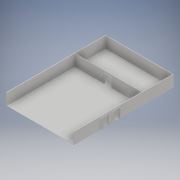
# Autodesk Inventor part: Top Office Layer
Saved by Autodesk Inventor 2017 (Build 210142000, 142)
## iProperties
Created: 2018-04-17
Part Number: Top Office Layer
Material: Generic
Document SubType Name: Modeling
Designer: landontracy
Density: 1 g/cm^3
Appearance: Default
Author: landontracy
Autodesk Inventor part; units mm, degrees
ref_plane "YZ Plane" through (0, 0, 0) normal (1, 0, 0) x (0, 1, 0)
ref_plane "XZ Plane" through (0, 0, 0) normal (0, 1, 0) x (-1, 0, 0)
ref_plane "XY Plane" through (0, 0, 0) normal (0, 0, 1) x (1, 0, 0)
sketch "Sketch1" plane through (0, 0, 0) normal (0, 0, 1) x (1, 0, 0)
  line L0 (-105.4358, -42.0697) -> (85.0642, -42.0697)
  line L1 (85.0642, -42.0697) -> (85.0642, 186.5303)
  line L2 (85.0642, 186.5303) -> (-105.4358, 186.5303)
  line L3 (-105.4358, 186.5303) -> (-105.4358, -42.0697)
  line L4 (-105.4358, -42.0697) -> (-156.2358, -42.0697)
  line L5 (-156.2358, -42.0697) -> (-156.2358, 237.3303)
  line L6 (-156.2358, 237.3303) -> (135.8642, 237.3303)
  line L7 (135.8642, 237.3303) -> (135.8642, -42.0697)
  line L8 (135.8642, -42.0697) -> (85.0642, -42.0697)
  point P0 (0, 0)
  dimension "d0" = 228.6
  dimension "d1" = 190.5
  dimension "d2" = 50.8
  dimension "d3" = 279.4
  dimension "d4" = 292.1
  constraints: 18 end point, 5 perpendicular, 2 horizontal, 2 parallel, 1 point on line
  measures "d0" distance of L0.end L1.end
  measures "d1" distance of L0.start L0.end
  measures "d2" distance of L0.start L4.end
  measures "d3" distance of L4.end L5.end
  measures "d4" distance of L5.end L6.end
extrude "Door Frame CR" add sketch "Sketch1" along normal mid plane 8.89 contours L4 L5 L6 L7 L8 L1 L2 L3
sketch "Sketch2" plane through (-156.2358, -42.0697, 4.445) normal (-1, 0, 0) x (0, 0, 1)
  line L0 (-8.89, 279.4) -> (-8.89, 0) projected
  line L1 (-8.89, 279.4) -> (0, 279.4)
  line L2 (0, 279.4) -> (0, 0)
  line L3 (0, 0) -> (-8.89, 0)
  line L4 (-8.89, 0) -> (-8.89, 279.4)
  point P0 (-4.445, 42.0697)
  constraints: 8 end point, 2 parallel, 1 horizontal, 1 perpendicular
extrude "Door Frame left Extruded" add sketch "Sketch2" along normal blind 685.8
sketch "Sketch4" plane through (135.8642, -42.0697, 4.445) normal (1, 0, 0) x (0, 0, -1)
  line L0 (0, 0) -> (0, 279.4) projected
  line L1 (8.89, 228.6) -> (8.89, 0) projected
  line L2 (0, 279.4) -> (8.89, 279.4)
  line L3 (8.89, 279.4) -> (8.89, 0)
  line L4 (8.89, 0) -> (0, 0)
  line L5 (0, 0) -> (0, 279.4)
  point P0 (4.445, 42.0697)
  constraints: 8 end point, 2 parallel, 1 horizontal, 1 perpendicular
extrude "Door Frame right Extruded" add sketch "Sketch4" along normal blind 685.8
sketch "Sketch5" plane through (0, 0, 4.445) normal (0, 0, 1) x (1, 0, 0)
  line L0 (-842.0358, 237.3303) -> (-842.0358, -42.0697) projected
  line L1 (821.6642, 237.3303) -> (821.6642, -42.0697) projected
  line L2 (-842.0358, -42.0697) -> (821.6642, -42.0697)
  line L3 (821.6642, -42.0697) -> (821.6642, -36.9897)
  line L4 (821.6642, -36.9897) -> (-842.0358, -36.9897)
  line L5 (-842.0358, -36.9897) -> (-842.0358, -42.0697)
  point P0 (0, 0)
  dimension "d11" = 5.08
  constraints: 8 end point, 2 parallel, 1 horizontal, 1 perpendicular, 1 point on line
  measures "d11" distance of L3.end L2.end
extrude "Floor" add sketch "Sketch5" along normal blind 762
sketch "Sketch7" plane through (-105.4358, -36.9897, 4.445) normal (0, 1, 0) x (1, 0, 0)
  line L0 (-736.6, 0) -> (0, 0) projected
  line L1 (-736.6, -762) -> (927.1, -762) projected
  line L2 (-736.6, 0) -> (-723.9, 0)
  line L3 (-723.9, 0) -> (-723.9, -749.3)
  line L4 (-723.9, -762) -> (-736.6, -762)
  line L5 (-736.6, -762) -> (-736.6, 0)
  line L6 (927.1, 8.89) -> (927.1, -762) projected
  line L7 (-723.9, -762) -> (927.1, -762)
  line L8 (927.1, -762) -> (927.1, -749.3)
  line L9 (914.4, -749.3) -> (-723.9, -749.3)
  line L10 (190.5, 0) -> (927.1, 0) projected
  line L11 (914.4, -749.3) -> (914.4, 0)
  line L12 (914.4, 0) -> (927.1, 0)
  line L13 (927.1, 0) -> (927.1, -749.3)
  point P0 (105.4358, 4.445)
  dimension "d21" = 12.7
  dimension "d55" = 1663.7
  constraints: 20 end point, 4 parallel, 3 point on line, 2 horizontal, 2 perpendicular
  measures "d21" distance of L11.end L12.end
  measures "d55" distance of L1.start L1.end
extrude "Walls" add sketch "Sketch7" along normal blind 274.6375
sketch "Door Frame" plane through (0, 0, 4.445) normal (0, 0, 1) x (1, 0, 0)
  line L0 (-105.4358, -36.9897) -> (-105.4358, 186.5303) projected
  line L1 (-105.4358, -36.9897) -> (-113.0558, -36.9897)
  line L2 (-113.0558, -36.9897) -> (-113.0558, 186.5303)
  line L3 (-105.4358, 186.5303) -> (-105.4358, -36.9897)
  line L4 (-105.4358, 186.5303) -> (85.0642, 186.5303) projected
  line L5 (92.6842, 185.3187) -> (92.6842, -36.9897)
  line L6 (92.6842, -36.9897) -> (85.0642, -36.9897)
  line L7 (85.0642, -36.9897) -> (85.0642, 186.5303)
  line L8 (-105.4358, 186.5303) -> (85.0642, 186.5303)
  line L9 (92.6842, 185.3187) -> (92.6842, 194.1503)
  line L10 (92.6842, 194.1503) -> (-113.0558, 194.1503)
  line L11 (-113.0558, 194.1503) -> (-113.0558, 186.5303)
  point P0 (0, 0)
  dimension "d27" = 7.62
  dimension "d28" = 7.62
  dimension "d29" = 7.62
  constraints: 20 end point, 4 parallel, 2 collinear, 2 horizontal, 2 perpendicular, 1 point on line
  measures "d27" distance between parallel lines of L10 L4
  measures "d28" distance between parallel lines of L5 L7
  measures "d29" distance between parallel lines of L0 L2
extrude "Door Fram ex" add sketch "Door Frame" along normal blind 7.9375
fillet "Dorr Fillet" radius 0.508 1 edges at (-113.0558, 194.1503, 8.4138)
fillet "Door Fillet" radius 0.508 1 edges at (92.6842, 194.1503, 8.4138)
sketch "Sketch9" plane through (0, 0, 4.445) normal (0, 0, -1) x (-1, 0, 0)
  line L0 (-85.0642, -36.9897) -> (-85.0642, -42.0697) projected
  line L1 (-85.0642, -36.9897) -> (105.4358, -36.9897)
  line L2 (105.4358, -36.9897) -> (105.4358, -42.0697)
  line L3 (105.4358, -42.0697) -> (-85.0642, -42.0697)
  line L4 (-85.0642, -42.0697) -> (-85.0642, -36.9897)
  point P0 (0, 0)
  constraints: 8 end point, 2 parallel, 1 horizontal, 1 perpendicular
extrude "Door floor" add sketch "Sketch9" along normal blind 8.89
sketch "Sketch13" plane through (808.9642, -36.9897, 753.745) normal (0, 0, -1) x (-1, 0, 0)
  line L0 (-12.7, -5.08) -> (-12.7, 274.6375) projected
  line L1 (-12.7, 31.9391) -> (1651, 31.9391)
  line L2 (1651, 31.9391) -> (1651, -1.0809)
  line L3 (1651, -1.0809) -> (-12.7, -1.0809)
  line L4 (-12.7, -1.0809) -> (-12.7, 31.9391)
  point P0 (808.9642, 36.9897)
  dimension "d36" = 33.02
  dimension "d42" = 37.0191
  constraints: 8 end point, 2 parallel, 1 horizontal, 1 perpendicular, 1 point on line
  measures "d36" distance of L1.end L2.end
  measures "d42" distance of L0.start L1.start
extrude "wall board middle" add sketch "Sketch13" along normal blind 2.54
sketch "Sketch14" plane through (808.9642, -36.9897, 4.445) normal (-1, 0, 0) x (0, 0, 1)
  line L0 (-8.89, -5.08) -> (-8.89, 274.32) projected
  line L1 (762, -5.08) -> (762, 274.6375) projected
  line L2 (-8.89, -5.08) -> (762, -5.08)
  line L3 (762, -5.08) -> (762, 31.877)
  line L4 (762, 31.877) -> (-8.89, 31.877)
  line L5 (-8.89, 31.877) -> (-8.89, -5.08)
  point P0 (-4.445, 36.9897)
  dimension "d39" = 36.957
  constraints: 8 end point, 2 parallel, 1 horizontal, 1 perpendicular, 1 point on line
  measures "d39" distance of L3.end L2.end
extrude "Wall board left" add sketch "Sketch14" along normal blind 2.54
sketch "Sketch16" plane through (-829.3358, -36.9897, 4.445) normal (1, 0, 0) x (0, 0, -1)
  line L0 (8.89, -5.08) -> (-762, -5.08) projected
  line L1 (8.89, 274.32) -> (8.89, -5.08) projected
  line L2 (-762, -5.08) -> (8.89, -5.08)
  line L3 (8.89, -5.08) -> (8.89, 31.9278)
  line L4 (8.89, 31.9278) -> (-762, 31.9278)
  line L5 (-762, 31.9278) -> (-762, -5.08)
  point P0 (4.445, 36.9897)
  dimension "d43" = 37.0078
  constraints: 8 end point, 2 parallel, 1 horizontal, 1 perpendicular, 1 point on line
  measures "d43" distance of L3.end L2.end
extrude "Wall board right" add sketch "Sketch16" along normal blind 2.54
sketch "Sketch20" plane through (0, 0, 4.445) normal (0, 0, 1) x (1, 0, 0)
  line L0 (821.6642, -42.0697) -> (821.6642, 237.3303) projected
  line L1 (821.6642, -42.0697) -> (821.6642, -5.0619)
  line L2 (-842.0358, -5.0619) -> (-842.0358, -42.0697)
  line L3 (-113.5303, -5.0619) -> (-113.5303, -42.0697)
  line L4 (92.92, -5.0619) -> (92.92, -42.0697)
  line L5 (821.6642, -5.0619) -> (92.92, -5.0619)
  line L6 (-113.5303, -5.0619) -> (-842.0358, -5.0619)
  line L7 (-842.0358, -42.0697) -> (-113.5303, -42.0697)
  line L8 (92.92, -42.0697) -> (821.6642, -42.0697)
  point P0 (0, 0)
  dimension "d47" = 37.0078
  constraints: 16 end point, 6 perpendicular, 5 parallel, 2 horizontal, 1 point on line
  measures "d47" distance of L1.end L1.start
extrude "Wall board door" add sketch "Sketch20" along normal blind 2.54
sketch "Sketch22" plane through (0, 0, -4.445) normal (0, 0, -1) x (-1, 0, 0)
  line L0 (-92.6842, -36.9897) -> (-92.6842, 193.6423) projected
  line L1 (-92.6842, -36.9897) -> (-92.6842, 193.6423)
  line L2 (113.0558, 193.6423) -> (113.0558, -36.9897) projected
  line L3 (-92.6842, 193.6423) -> (113.0558, 193.6423)
  line L4 (113.0558, 193.6423) -> (113.0558, -36.9897)
  line L5 (826.7958, -36.9897) -> (-806.4242, -36.9897) projected
  line L6 (-85.0642, 186.5303) -> (-85.0642, -36.9897) projected
  line L7 (-92.6842, -36.9897) -> (-85.0642, -36.9897)
  line L8 (105.4358, 186.5303) -> (-85.0642, 186.5303) projected
  line L9 (-85.0642, -36.9897) -> (-85.0642, 186.5303)
  line L10 (105.4358, -36.9897) -> (105.4358, 186.5303) projected
  line L11 (-85.0642, 186.5303) -> (105.4358, 186.5303)
  line L12 (105.4358, 186.5303) -> (105.4358, -36.9897)
  line L13 (105.4358, -36.9897) -> (113.0558, -36.9897)
  point P0 (0, 0)
  constraints: 16 end point, 5 perpendicular, 2 collinear, 1 horizontal, 1 point on line
extrude "Door mid" add sketch "Sketch22" along normal blind 8.89 contours L0 L3 L2 L5 L10 L8 L6
sketch "Sketch23" plane through (0, 0, -4.445) normal (0, 0, -1) x (-1, 0, 0)
  line L0 (-806.4242, -5.1127) -> (-806.4242, -36.9897) projected
  line L1 (-821.6642, 237.3303) -> (-806.4242, 237.3303)
  line L2 (-806.4242, 237.3303) -> (-806.4242, -36.9897)
  line L3 (-806.4242, -36.9897) -> (-821.6642, -36.9897)
  line L4 (-821.6642, -36.9897) -> (-821.6642, 237.3303)
  point P0 (0, 0)
  constraints: 8 end point, 2 parallel, 1 horizontal, 1 perpendicular
extrude "Main wall left" add sketch "Sketch23" along normal blind 1663.7
sketch "Sketch24" plane through (0, 0, -4.445) normal (0, 0, -1) x (-1, 0, 0)
  line L0 (829.3358, 237.6478) -> (842.0358, 237.6478) projected
  line L1 (826.7958, -36.9897) -> (826.7958, -5.0619) projected
  line L2 (842.0358, 237.6478) -> (826.7958, 237.6478)
  line L3 (826.7958, 237.6478) -> (826.7958, -36.9897)
  line L4 (826.7958, -36.9897) -> (842.0358, -36.9897)
  line L5 (842.0358, -36.9897) -> (842.0358, 237.6478)
  point P0 (0, 0)
  constraints: 8 end point, 2 parallel, 1 horizontal, 1 perpendicular
extrude "Main wall right" add sketch "Sketch24" along normal blind 1663.7
sketch "Sketch26" plane through (0, 0, -4.445) normal (0, 0, -1) x (-1, 0, 0)
  line L0 (-821.6642, -42.0697) -> (-821.6642, -36.9897) projected
  line L1 (842.0358, -42.0697) -> (-821.6642, -42.0697) projected
  line L2 (-821.6642, -36.9897) -> (842.0358, -36.9897)
  line L3 (842.0358, -36.9897) -> (842.0358, -42.0697)
  line L4 (842.0358, -42.0697) -> (-821.6642, -42.0697)
  line L5 (-821.6642, -42.0697) -> (-821.6642, -36.9897)
  point P0 (0, 0)
  constraints: 8 end point, 2 parallel, 1 horizontal, 1 perpendicular
extrude "prob the floor" add sketch "Sketch26" along normal blind 1663.7
sketch "Sketch27" plane through (0, 0, -4.445) normal (0, 0, -1) x (-1, 0, 0)
  line L0 (842.0358, -42.0697) -> (842.0358, -5.0507)
  line L1 (-821.6642, -5.0507) -> (-821.6642, -5.1127)
  line L2 (-92.92, -5.0619) -> (-92.92, -36.9897) projected
  line L3 (113.0558, -5.0507) -> (113.0558, -42.0697)
  line L4 (842.0358, -5.0507) -> (113.0558, -5.0507)
  line L5 (-92.6842, -5.0507) -> (-806.4242, -5.0507)
  line L6 (-806.4242, -42.0697) -> (-92.92, -42.0697)
  line L7 (113.0558, -42.0697) -> (842.0358, -42.0697)
  line L8 (-806.4242, -5.1127) -> (-806.4242, -42.0697)
  line L9 (-806.4242, -5.1127) -> (-806.4242, -5.0507)
  line L10 (-93.1904, -5.0507) -> (-93.1904, -42.4087)
  point P0 (0, 0)
  dimension "d60" = 37.0191
  constraints: 20 end point, 5 parallel, 3 perpendicular, 2 horizontal, 1 point on line, 1 vertical
  measures "d60" distance of L0.end L0.start
extrude "wall board front main 1" add sketch "Sketch27" along normal blind 2.54 contours L7 L3 L4 L0
sketch "Sketch28" plane through (0, 0, -4.445) normal (0, 0, -1) x (-1, 0, 0)
  line L0 (-806.4242, -36.9897) -> (-92.92, -36.9897) projected
  line L1 (-92.8218, -0.013) -> (-806.4242, -0.013)
  line L2 (-806.4242, -0.013) -> (-806.4242, -36.9897)
  line L3 (-806.4242, -36.9897) -> (-92.8218, -36.9897)
  line L4 (-92.8218, -36.9897) -> (-92.8218, -0.013)
  point P0 (-808.9642, -5.0507)
  point P1 (-92.92, -5.0619)
  point P2 (-92.6842, -36.9897)
  constraints: 8 end point, 2 parallel, 1 horizontal, 1 perpendicular
extrude "wall board front main 2" add sketch "Sketch28" along normal blind 2.54
sketch "Sketch30" plane through (806.4242, -36.9897, -1668.145) normal (-1, 0, 0) x (0, 0, 1)
  line L0 (1661.16, 0) -> (1661.16, 36.9767) projected
  line L1 (0, 0) -> (0, 274.32) projected
  line L2 (1661.16, 36.9767) -> (0, 36.9767)
  line L3 (0, 36.9767) -> (0, 0)
  line L4 (0, 0) -> (1661.16, 0)
  line L5 (1661.16, 0) -> (1661.16, 36.9767)
  point P0 (1668.145, 36.9897)
  constraints: 8 end point, 2 parallel, 1 horizontal, 1 perpendicular
extrude "wall board front left" add sketch "Sketch30" along normal blind 2.54
sketch "Sketch31" plane through (-826.7958, -36.9897, -1668.145) normal (1, 0, 0) x (0, 0, -1)
  line L0 (-1661.16, 31.9391) -> (-1661.16, 0) projected
  line L1 (0, 274.6375) -> (0, 0) projected
  line L2 (-1661.16, 31.9391) -> (0, 31.9391)
  line L3 (0, 31.9391) -> (0, 0)
  line L4 (0, 0) -> (-1661.16, 0)
  line L5 (-1661.16, 0) -> (-1661.16, 31.9391)
  point P0 (-1668.145, 36.9897)
  constraints: 8 end point, 2 parallel, 1 horizontal, 1 perpendicular
extrude "wall board front right" add sketch "Sketch31" along normal blind 2.54
sketch "Sketch32" plane through (-826.7958, 237.6478, -4.445) normal (1, 0, 0) x (0, 0, -1)
  line L0 (-755.65, -242.7097) -> (-8.89, -242.7097) projected
  line L1 (557.2999, -274.6375) -> (557.2999, 4.7625)
  line L2 (557.2999, 4.7625) -> (747.7999, 4.7625)
  line L3 (747.7999, 4.7625) -> (747.7999, -274.6375)
  line L4 (832.2959, -274.6375) -> (1022.7959, -274.6375)
  line L5 (1022.7959, -274.6375) -> (1022.7959, 4.7625)
  line L6 (1022.7959, 4.7625) -> (832.2959, 4.7625)
  line L7 (832.2959, 4.7625) -> (832.2959, -274.6375)
  line L8 (557.2999, -274.6375) -> (747.7999, -274.6375)
  line L9 (1663.7, -274.6375) -> (2.54, -274.6375) projected
  point P0 (-4.445, -237.6478)
  dimension "d69" = 190.5
  dimension "d70" = 190.5
  dimension "d71" = 279.4
  dimension "d72" = 279.4
  constraints: 16 end point, 3 parallel, 3 point on line, 2 collinear, 2 perpendicular, 1 horizontal
  measures "d69" distance of L3.end L1.start
  measures "d70" distance of L4.start L4.end
  measures "d71" distance of L1.start L1.end
  measures "d72" distance of L4.end L5.end
extrude "Right doors" cut sketch "Sketch32" along normal mid plane 76.2
sketch "Sketch33" plane through (0, 0, -4.445) normal (0, 0, -1) x (-1, 0, 0)
  line L0 (113.0558, 193.6423) -> (113.0558, 237.3303)
  line L1 (-806.4242, 237.3303) -> (826.7958, 237.3303) projected
  point P0 (0, 0)
  dimension "d77" = 43.688
  constraints: 2 end point, 1 point on line, 1 vertical
  measures "d77" distance of L0.start L0.end
sketch "Sketch34" plane through (-826.7958, -5.0507, -561.7449) normal (0, 0, -1) x (-1, 0, 0)
  line L0 (15.24, -37.0191) -> (15.24, 242.6984) projected
  line L1 (0, 0) -> (0, 242.3809) projected
  line L2 (15.24, 242.6984) -> (0, 242.6984)
  line L3 (0, 242.6984) -> (0, 199.0104)
  line L4 (0, 199.0104) -> (15.24, 199.0104)
  line L5 (15.24, 199.0104) -> (15.24, 242.6984)
  point P0 (-826.7958, 5.0507)
  dimension "d78" = 43.688
  constraints: 8 end point, 2 parallel, 1 horizontal, 1 perpendicular, 1 point on line
  measures "d78" distance of L3.end L2.end
extrude "Right doors head" add sketch "Sketch34" along normal blind 517.525
sketch "Sketch35" plane through (0, 0, -13.335) normal (0, 0, -1) x (-1, 0, 0)
  line L0 (-84.9391, 54.3094) -> (-92.6842, 54.3094)
  line L1 (-92.6842, -36.9897) -> (-92.6842, 193.6423) projected
  point P0 (0, 0)
  dimension "d81" = 7.7451
  constraints: 2 end point, 1 horizontal, 1 point on line
  measures "d81" distance of L0.start L0.end
sketch "Sketch36" plane through (-826.7958, 237.6478, -4.445) normal (1, 0, 0) x (0, 0, -1)
  line L0 (557.2999, -274.6375) -> (549.5548, -274.6375)
  line L1 (1022.7959, -274.6375) -> (1022.7959, -43.688) projected
  line L2 (1022.7959, -274.6375) -> (1030.5409, -274.6375)
  line L3 (557.2999, -43.688) -> (747.7999, -43.688) projected
  line L4 (549.5548, -35.9429) -> (549.5548, -274.6375)
  line L5 (557.2999, -274.6375) -> (747.7999, -274.6375) projected
  line L6 (557.2999, -43.688) -> (557.2999, -274.6375)
  line L7 (557.2999, -43.688) -> (747.7999, -43.688)
  line L8 (747.7999, -274.6375) -> (747.7999, -43.688) projected
  line L9 (747.7999, -43.688) -> (747.7999, -274.6375)
  line L10 (557.2999, -43.688) -> (557.2999, -274.6375) projected
  line L11 (832.2959, -43.688) -> (832.2959, -274.6375) projected
  line L12 (832.2959, -274.6375) -> (832.2959, -43.688)
  line L13 (832.2959, -43.688) -> (1022.7959, -43.688)
  line L14 (1022.7959, -43.688) -> (1022.7959, -274.6375)
  line L15 (-770.89, -279.7175) -> (1663.7, -279.7175) projected
  line L16 (755.545, -127.9526) -> (755.545, -35.9429)
  line L17 (755.545, -127.9526) -> (755.545, -274.6375)
  line L18 (824.5508, -127.9526) -> (824.5508, -35.9429)
  line L19 (824.5508, -127.9526) -> (824.5508, -274.6375)
  line L20 (1022.7959, -274.6375) -> (1030.5409, -274.6375)
  line L21 (1030.5409, -274.6375) -> (1022.7959, -274.6375)
  line L22 (824.5508, -274.6375) -> (832.2959, -274.6375)
  line L23 (832.2959, -274.6375) -> (824.5508, -274.6375)
  line L24 (755.545, -274.6375) -> (747.7999, -274.6375)
  line L25 (549.5548, -274.6375) -> (557.2999, -274.6375)
  line L26 (747.7999, -274.6375) -> (755.545, -274.6375)
  line L27 (1030.5409, -35.9429) -> (824.5508, -35.9429)
  line L28 (755.545, -35.9429) -> (549.5548, -35.9429)
  line L29 (1030.5409, -127.9526) -> (1030.5409, -35.9429)
  line L30 (1030.5409, -127.9526) -> (1030.5409, -274.6375)
  point P0 (-4.445, -237.6478)
  dimension "d82" = 7.7451
  constraints: 49 end point, 15 perpendicular, 8 parallel, 6 horizontal, 2 point on line, 2 vertical, 1 collinear
  measures "d82" distance of L0.start L0.end
extrude "Right doors frame mid" add sketch "Sketch36" along normal blind 7.62 contours L0 L4 L28 L16 L17 L24 L8 L3 L6 | L1 L13 L11 L22 L19 L18 L27 L29 L30 L2
sketch "Sketch38" plane through (-842.0358, -42.0697, 4.445) normal (-1, 0, 0) x (0, 0, 1)
  line L0 (-1039.4309, 5.08) -> (-1039.4309, 243.7746) projected
  line L1 (-1039.4309, 5.08) -> (-1039.4309, 243.7746)
  line L2 (-1039.4309, 243.7746) -> (-833.4408, 243.7746) projected
  line L3 (-1039.4309, 243.7746) -> (-833.4408, 243.7746)
  line L4 (-833.4408, 243.7746) -> (-833.4408, 5.08) projected
  line L5 (-833.4408, 243.7746) -> (-833.4408, 5.08)
  line L6 (-841.1859, 236.0295) -> (-841.1859, 5.08) projected
  line L7 (-833.4408, 5.08) -> (-841.1859, 5.08)
  line L8 (-841.1859, 5.08) -> (-841.1859, 235.751)
  line L9 (-841.1859, 235.751) -> (-1030.9904, 235.751)
  line L10 (-1030.9904, 235.751) -> (-1030.9904, 5.08)
  line L11 (-11.43, 5.08) -> (-1672.59, 5.08) projected
  line L12 (-1039.4309, 5.08) -> (-1030.9904, 5.08)
  line L13 (-1672.59, 0) -> (762, 0) projected
  line L14 (-764.435, 5.08) -> (-764.435, 243.7746) projected
  line L15 (-833.4408, 5.08) -> (-764.435, 5.08) projected
  line L16 (-764.435, 243.7746) -> (-764.435, 5.08)
  line L17 (-566.1899, 5.08) -> (-756.6899, 5.08) projected
  line L18 (-764.435, 5.08) -> (-756.6899, 5.08)
  line L19 (-756.6899, 5.08) -> (-756.6899, 236.0295) projected
  line L20 (-756.6899, 5.08) -> (-756.6899, 236.0295)
  line L21 (-566.1899, 236.0295) -> (-566.1899, 5.08) projected
  line L22 (-756.6899, 236.0295) -> (-566.1899, 236.0295)
  line L23 (-566.1899, 236.0295) -> (-566.1899, 5.08)
  line L24 (-558.4448, 243.7746) -> (-558.4448, 5.08) projected
  line L25 (-566.1899, 5.08) -> (-558.4448, 5.08)
  line L26 (-558.4448, 5.08) -> (-558.4448, 243.7746)
  line L27 (-558.4448, 243.7746) -> (-764.435, 243.7746)
  point P0 (-4.445, 42.0697)
  constraints: 32 end point, 9 perpendicular, 4 collinear, 2 vertical, 1 parallel, 3 other
extrude "right doors frame into" add sketch "Sketch38" along normal blind 7.62 contours L0 L2 L4 L7 L6 L9 L10 L11 | L11 L21 L22 L19 L14 L27 L24
equation "\"d53\" = d55"
equation "\"d56\" = d55"
equation "\"d58\" = d55"
equation "\"d60\" = d42"
equation "\"d69\" = d1"
equation "\"d70\" = d1"
equation "\"d71\" = d3"
equation "\"d72\" = d3"
equation "\"d78\" = d77"
equation "\"d82\" = d81"
body "Solid1"
